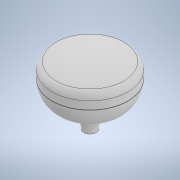
# Autodesk Inventor part: Рукоятка
Saved by Autodesk Inventor 2021 (Build 250183000, 183)
## iProperties
Created: 2021-04-19
Part Number: Рукоятка
Material: Типовые
Document SubType Name: Modeling
Designer: Данил
Density: 1 g/cm^3
Appearance: По умолчанию
Author: Данил
Autodesk Inventor part; units mm, degrees
ref_plane "YZ Plane" through (0, 0, 0) normal (1, 0, 0) x (0, 1, 0)
ref_plane "XZ Plane" through (0, 0, 0) normal (0, 1, 0) x (-1, 0, 0)
ref_plane "XY Plane" through (0, 0, 0) normal (0, 0, 1) x (1, 0, 0)
sketch "Эскиз1" plane through (0, 0, 0) normal (0, 0, 1) x (1, 0, 0)
  line L0 (0, 40) -> (0, -40)
  arc A0 (45, 26.1438) -> (0, 40) centre (0, -40) ccw
  line L1 (45, 26.1438) -> (45, 11.1438)
  arc A1 (24.5531, -16.2967) -> (45, 11.1438) centre (15.0168, 12.1473) ccw
  arc A2 (24.5531, -16.2967) -> (7.5, -40) centre (32.5, -40) ccw
  line L2 (0, -40) -> (7.5, -40)
  point P0 (0, 0)
  point P1 (0, 0)
  dimension "d0" = 80
  dimension "d1" = 90
  dimension "d2" = 15
  dimension "d3" = 15
  dimension "d4" = 30
  dimension "d5" = 25
  constraints: 6 end point, 6 point on circle, 3 centre point, 2 coincident, 2 horizontal alignment, 2 line through centre, 2 vertical, 1 horizontal, 1 midpoint, 1 tangent
  measures "d0" distance of L0.start L0.end
  measures "d1" diameter of L1 L0
  measures "d2" distance of L1.start L1.end
  measures "d3" diameter of L2.end L0
  measures "d4" radius of A1
  measures "d5" radius of A2
revolve "Вращение1" add sketch "Эскиз1" angle 360 about axis through (0, 40, 0) along (0, -1, 0)
fillet "Сопряжение1" radius 10 2 edges at (-45, 26.1438, 0) (-45, 11.1438, 0)
sketch "Эскиз2" plane through (0, -40, 0) normal (0, -1, 0) x (1, 0, 0)
  circle A0 centre (0, 0) radius 7.5 projected
  point P0 (0, 0)
  constraints: 1 coincident
hole "Отверстие1" at (0, -40, 0) direction (0, 1, 0) diameter 8.9175 depth 21 tip angle 120 thread size "M10x1" class "6H" standard "ISO Metric profile"
